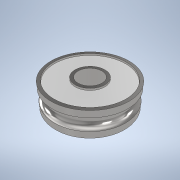
# Autodesk Inventor part: U-подшипник
Saved by Autodesk Inventor 2021.1 (Build 251245010, 245A)
## iProperties
Created: 2023-09-11
Part Number: U-подшипник
Material: Типовые
Document SubType Name: Modeling
Designer: Andrew
Density: 1 g/cm^3
Appearance: По умолчанию
Author: Andrew
Autodesk Inventor part; units mm, degrees
ref_plane "YZ Plane" through (0, 0, 0) normal (1, 0, 0) x (0, 1, 0)
sketch "Эскиз1" plane through (0, 0, 0) normal (0, 1, 0) x (-1, 0, 0)
  circle A0 centre (0, 0) radius 2
  circle A1 centre (0, 0) radius 6.5
  dimension "d1" = 4
  dimension "d2" = 13
  constraints: 2 centre point, 2 coincident
  measures "d1" diameter of A0
  measures "d2" diameter of A1
extrude "Выдавливание1" add sketch "Эскиз1" along normal blind 4
sketch "Эскиз2" plane through (0, 4, 0) normal (0, 1, 0) x (1, 0, 0)
  circle A0 centre (0, 0) radius 2 projected
  circle A1 centre (0, 0) radius 2.5
  circle A2 centre (0, 0) radius 6
  dimension "d5" = 5
  dimension "d6" = 12
  constraints: 2 centre point, 2 coincident
  measures "d5" diameter of A1
  measures "d6" diameter of A2
extrude "Выдавливание2" cut sketch "Эскиз2" against normal blind 0.3 contours A2
sketch "Эскиз3" plane through (0, 0, 0) normal (0, -1, 0) x (1, 0, 0)
  circle A0 centre (0, 0) radius 2.5
  circle A1 centre (0, 0) radius 6
  dimension "d9" = 5
  dimension "d10" = 12
  constraints: 2 centre point, 2 coincident
  measures "d9" diameter of A0
  measures "d10" diameter of A1
extrude "Выдавливание3" cut sketch "Эскиз3" against normal blind 0.3
ref_plane "РабПлоскость1" through (0, 2, 0) normal (0, 1, 0) x (1, 0, 0)
sketch "Эскиз4" plane through (0, 2, 0) normal (0, 1, 0) x (1, 0, 0)
  circle A0 centre (0, 0) radius 6.5
  dimension "d13" = 13
  constraints: 1 centre point, 1 coincident
  measures "d13" diameter of A0
ref_plane "РабПлоскость2" through (0, 0, 0) normal (0, 0, 1) x (1, 0, 0)
sketch "Эскиз6" plane through (0, 0, 0) normal (0, 0, 1) x (1, 0, 0)
  line L0 (-6.5, 0) -> (-6.5, 4) projected
  circle A0 centre (-6.5, 2) radius 1
  line L1 (0, -0.8) -> (0, 4.8) projected
  point P0 (0, 0)
  dimension "d15" = 2
  constraints: 1 centre point, 1 midpoint
  measures "d15" diameter of A0
revolve "Вращение1" cut sketch "Эскиз6" angle 360 about axis through (0, -10, 0) along (0, 1, 0)
